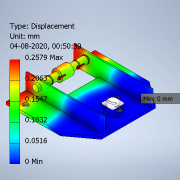
# Autodesk Inventor part: base for ball scew -bolt
Saved by Autodesk Inventor 2020 (Build 240168000, 168)
## iProperties
Created: 2020-07-27
Part Number: base for ball scew -bolt
Material: Steel, Mild
Document SubType Name: Modeling
Designer: Vikki
Mass: 4960.92 g
Surface Area: 1915.07 cm^2
Volume: 631.964 cm^3
Density: 7.85 g/cm^3
Appearance: Semi-Polished
Author: Vikki
Autodesk Inventor part; units mm, degrees
ref_plane "Work Plane1" through (0, 0, 4950) normal (0, 0, 1) x (1, 0, 0)
sketch "Sketch1" plane through (0, 0, 4950) normal (0, 0, 1) x (1, 0, 0)
  circle A0 centre (180, 0) radius 12.5 projected
  circle A1 centre (180, 17.5) radius 2 projected
  circle A2 centre (197.5, 0) radius 2 projected
  circle A3 centre (162.5, 0) radius 2 projected
  circle A4 centre (180, -17.5) radius 2 projected
  line L0 (40, 182.7) -> (-40, 182.7) projected
  line L1 (-40, 182.7) -> (-40, -182.7) projected
  line L2 (-40, -182.7) -> (40, -182.7) projected
  line L3 (40, -182.7) -> (40, -50) projected
  line L4 (40, -50) -> (260, -50) projected
  line L5 (260, -50) -> (260, 50) projected
  line L6 (260, 50) -> (40, 50) projected
  line L7 (40, 50) -> (40, 182.7) projected
  circle A5 centre (0, 120) radius 8 projected
  circle A6 centre (0, -120) radius 8 projected
  circle A7 centre (0, -120) radius 8.5
  circle A8 centre (0, 120) radius 8.5
  line L8 (40, 182.7) -> (40, -182.7)
  line L9 (40, -182.7) -> (80, -182.7)
  line L10 (80, -182.7) -> (80, 182.7)
  line L11 (80, 182.7) -> (40, 182.7)
  line L12 (-40, 75) -> (40, 75)
  line L13 (40, 75) -> (40, -75)
  line L14 (40, -75) -> (-40, -75)
  line L15 (80, 182.7) -> (260, 50)
  line L16 (260, -50) -> (80, -182.7)
  line L17 (80, -142.7) -> (-40, -142.7)
  line L18 (-40, 142.7) -> (80, 142.7)
  line L19 (80, 142.7) -> (134.2577, 142.7)
  line L20 (80, -142.7) -> (134.2577, -142.7)
  line L21 (210, 86.8611) -> (210, -86.8611)
  point P0 (0, 0)
  point P1 (40, 75)
  dimension "d0" = 17
  dimension "d1" = 17
  dimension "d2" = 40
  dimension "d3" = 40
  dimension "d4" = 75
  dimension "d5" = 75
  dimension "d23" = 40
  dimension "d24" = 40
  dimension "d25" = 50
  constraints: 28 end point, 10 point on line, 5 perpendicular, 4 parallel, 2 centre point, 2 coincident, 2 horizontal, 1 vertical
  measures "d0" diameter of A7
  measures "d1" diameter of A8
  measures "d2" distance of L2.end L9.end
  measures "d3" distance from line of point (0, 0) L13
  measures "d4" distance from line of point (0, 0) L14
  measures "d5" distance from line of L12 point (0, 0)
  measures "d23" distance between parallel lines of L17 L2
  measures "d24" distance between parallel lines of L0 L18
  measures "d25" distance between parallel lines of L21 L5
extrude "Extrusion1" add sketch "Sketch1" along normal blind 8 contours A0 | A1 | A2 | A3 | A4 | L18 L10 L6 L7 | L7 L12 L1 L18 | L19 L15 L21 L6 L10 | L6 L10 L4 L8 | L6 L21 L4 L10 | L14 L3 L17 L1 | L4 L10 L17 L3 | L4 L21 L16 L20 L10
sketch "Sketch2" plane through (0, 0, 4958) normal (0, 0, 1) x (1, 0, 0)
  line L0 (-40, 75) -> (40, 75) projected
  line L1 (-40, 75) -> (40, 75)
  line L2 (40, 75) -> (40, 79)
  line L3 (40, 79) -> (-40, 79)
  line L4 (-40, 79) -> (-40, 75)
  line L5 (40, -75) -> (-40, -75) projected
  line L6 (40, -75) -> (-40, -75)
  line L7 (-40, -75) -> (-40, -79)
  line L8 (-40, -79) -> (40, -79)
  line L9 (40, -79) -> (40, -75)
  line L10 (-20, 79) -> (-20, -79)
  line L11 (20, -79) -> (20, 79)
  point P0 (0, 0)
  point P1 (20, 75)
  point P2 (-20, 75)
  point P3 (20, -75)
  point P4 (-20, -75)
  dimension "d8" = 4
  dimension "d9" = 4
  dimension "d12" = 20
  dimension "d13" = 20
  constraints: 20 end point, 6 equal length, 4 perpendicular, 4 point on line
  measures "d8" distance of L0.end L2.end
  measures "d9" distance of L8.end L5.start
  measures "d12" distance from line of L10 point (0, 0)
  measures "d13" distance from line of L11 point (0, 0)
extrude "Extrusion2" add sketch "Sketch2" along normal blind 50 contours L10 L3 L11 L0 | L5 L11 L8 L10
sketch "Sketch3" plane through (-40, -75, 4950) normal (0, 1, 0) x (1, 0, 0)
  circle A0 centre (40, -38) radius 10.5
  line L0 (60, -58) -> (20, -58) projected
  line L1 (20, -8) -> (20, -58) projected
  point P0 (40, 4950)
  dimension "d16" = 21
  dimension "d17" = 20
  dimension "d18" = 20
  constraints: 1 centre point
  measures "d16" diameter of A0
  measures "d17" distance from line of L0 A0.centre
  measures "d18" distance from line of L1 A0.centre
extrude "Extrusion3" add sketch "Sketch3" along normal blind 163 and the other way blind 13
sketch "Sketch4" plane through (0, 0, 4958) normal (0, 0, 1) x (1, 0, 0)
  circle A0 centre (160, 17.5) radius 2 projected
  circle A1 centre (177.5, 0) radius 2 projected
  circle A2 centre (0, -120) radius 8 projected
  circle A3 centre (142.5, 0) radius 2 projected
  circle A4 centre (160, -17.5) radius 2 projected
  circle A5 centre (0, 120) radius 8 projected
  line L0 (30, 157.3) -> (30, 182.7) projected
  line L1 (40, 182.7) -> (30, 182.7) projected
  line L2 (40, 50) -> (40, 182.7) projected
  line L3 (260, 50) -> (40, 50) projected
  line L4 (260, -50) -> (260, 50) projected
  line L5 (40, -50) -> (260, -50) projected
  line L6 (40, -182.7) -> (40, -50) projected
  line L7 (30, -182.7) -> (40, -182.7) projected
  line L8 (30, -182.7) -> (30, -157.3) projected
  line L9 (30, -157.3) -> (-30, -157.3) projected
  line L10 (-30, -157.3) -> (-30, -182.7) projected
  line L11 (-40, -182.7) -> (-30, -182.7) projected
  line L12 (-40, 182.7) -> (-40, -182.7) projected
  line L13 (-30, 182.7) -> (-40, 182.7) projected
  line L14 (-30, 182.7) -> (-30, 157.3) projected
  line L15 (-30, 157.3) -> (30, 157.3) projected
  line L16 (250, 25.4) -> (224.6, 25.4) projected
  line L17 (224.6, 25.4) -> (224.6, -25.4) projected
  line L18 (224.6, -25.4) -> (250, -25.4) projected
  line L19 (250, -25.4) -> (250, 25.4) projected
  circle A6 centre (160, 0) radius 10 projected
  point P0 (0, 0)
extrude "Extrusion4" cut sketch "Sketch4" against normal up to surface (8 mm away) contours A0 | A1 | A3 | A4
sketch "Sketch5" plane through (0, 0, 4958) normal (0, 0, 1) x (1, 0, 0)
  circle A0 centre (160, 0) radius 7.5 projected
  circle A1 centre (160, 0) radius 8.25
  point P0 (0, 0)
  dimension "d28" = 16.5
  constraints: 1 centre point, 1 coincident
  measures "d28" diameter of A1
extrude "Extrusion5" cut sketch "Sketch5" against normal blind 10 contours A0 | A1
sketch "Sketch6" plane through (0, 0, 4950) normal (0, 0, -1) x (-1, 0, 0)
  circle A0 centre (-142.5, 0) radius 2 projected
  circle A1 centre (-177.5, 0) radius 2 projected
  circle A2 centre (-160, 17.5) radius 2 projected
  circle A3 centre (-160, -17.5) radius 2 projected
  line L0 (-134.2577, 142.7) -> (40, 142.7) projected
  line L1 (-210, 86.8611) -> (-134.2577, 142.7) projected
  line L2 (-210, -86.8611) -> (-210, 86.8611) projected
  line L3 (-134.2577, -142.7) -> (-210, -86.8611) projected
  line L4 (40, -142.7) -> (-134.2577, -142.7) projected
  line L5 (40, -75) -> (40, -142.7) projected
  line L6 (-40, -75) -> (40, -75) projected
  line L7 (-40, 75) -> (-40, -75) projected
  line L8 (40, 75) -> (-40, 75) projected
  line L9 (40, 142.7) -> (40, 75) projected
  circle A4 centre (0, -120) radius 8.5 projected
  circle A5 centre (0, 120) radius 8.5 projected
  circle A6 centre (-160, 0) radius 8.25 projected
  circle A7 centre (-160, 0) radius 22.5
  point P0 (0, 0)
  dimension "d31" = 45
  constraints: 1 centre point, 1 coincident
  measures "d31" diameter of A7
extrude "Extrusion6" add sketch "Sketch6" along normal blind 4 contours A7
sketch "Sketch7" plane through (160, 0, 4946) normal (0, 0, -1) x (-1, 0, 0)
  circle A0 centre (0, 0) radius 22.5 projected
  circle A1 centre (0, 0) radius 12.5
  circle A2 centre (0, 0) radius 9
  point P0 (160, 0)
  dimension "d34" = 25
  dimension "d47" = 18
  constraints: 2 centre point, 2 coincident
  measures "d34" diameter of A1
  measures "d47" diameter of A2
extrude "Extrusion7" add sketch "Sketch7" along normal blind 40 contours A1
sketch "Sketch9" plane through (0, 0, 5008) normal (0, 0, 1) x (1, 0, 0)
  circle A0 centre (160, 0) radius 8.25 construction
  circle A1 centre (142.5, 0) radius 2 construction
  circle A2 centre (177.5, 0) radius 2 construction
  circle A3 centre (160, 17.5) radius 2 construction
  circle A4 centre (160, -17.5) radius 2 construction
  line L0 (20, 79) -> (20, 75) projected
  line L1 (20, 75) -> (40, 75) projected
  line L2 (40, 75) -> (40, -75) projected
  line L3 (40, -75) -> (20, -75) projected
  line L4 (20, -75) -> (20, -79) projected
  line L5 (20, -79) -> (-20, -79) projected
  line L6 (-20, -79) -> (-20, -75) projected
  line L7 (-20, -75) -> (-40, -75) projected
  line L8 (-40, -75) -> (-40, -142.7) projected
  line L9 (-40, -142.7) -> (134.2577, -142.7) projected
  line L10 (134.2577, -142.7) -> (210, -86.8611) projected
  line L11 (210, -86.8611) -> (210, 86.8611) projected
  line L12 (210, 86.8611) -> (134.2577, 142.7) projected
  line L13 (134.2577, 142.7) -> (-40, 142.7) projected
  line L14 (-40, 142.7) -> (-40, 75) projected
  line L15 (-40, 75) -> (-20, 75) projected
  line L16 (-20, 75) -> (-20, 79) projected
  line L17 (-20, 79) -> (20, 79) projected
  circle A5 centre (0, -120) radius 8.5 projected
  circle A6 centre (0, 120) radius 8.5 projected
  circle A7 centre (160, 0) radius 12.5 projected
  circle A8 centre (160, 0) radius 9
  line L18 (20, -75) -> (-20, -75) projected
  line L19 (-20, 75) -> (20, 75) projected
  point P0 (0, 0)
  dimension "d37" = 18
  constraints: 1 centre point, 1 coincident
  measures "d37" diameter of A8
extrude "Extrusion8" [suppressed]
sketch "Sketch10" plane through (0, 0, 5012) normal (0, 0, 1) x (1, 0, 0)
  circle A0 centre (120, -75) radius 6
  circle A1 centre (90, 0) radius 6
  circle A2 centre (120, 75) radius 6
  circle A3 centre (160, 0) radius 12.5 projected
  point P0 (0, 0)
  dimension "d40" = 70
  dimension "d41" = 75
  dimension "d42" = 75
  dimension "d43" = 40
  dimension "d44" = 12
  constraints: 3 centre point, 2 equal radius, 1 horizontal alignment, 1 vertical alignment
  measures "d40" distance of A3.centre A1.centre
  measures "d41" vertical distance of A0.centre A3.centre
  measures "d42" vertical distance of A2.centre A3.centre
  measures "d43" horizontal distance of A3.centre A0.centre
  measures "d44" diameter of A0
extrude "Extrusion9" [suppressed]
sketch "Sketch11" plane through (20, -79, 4958) normal (1, 0, 0) x (0, 0, -1)
  line L0 (0, 4) -> (0, 0) projected
  line L1 (0, 4) -> (-50, 4) projected
  line L2 (-50, 0) -> (-50, 4) projected
  line L3 (0, 0) -> (-50, 0) projected
  line L4 (0, 158) -> (0, 154) projected
  line L5 (0, 158) -> (-50, 158) projected
  line L6 (-50, 154) -> (-50, 158) projected
  line L7 (0, 154) -> (-50, 154) projected
  point P0 (4958, 79)
extrude "Extrusion10" add sketch "Sketch11" along normal blind 190
sketch "Sketch12" plane through (-20, -79, 4958) normal (-1, 0, 0) x (0, 0, 1)
  line L0 (0, 154) -> (0, 158) projected
  line L1 (0, 154) -> (50, 154) projected
  line L2 (50, 158) -> (50, 154) projected
  line L3 (0, 158) -> (50, 158) projected
  line L4 (0, 0) -> (0, 4) projected
  line L5 (0, 0) -> (50, 0) projected
  line L6 (50, 4) -> (50, 0) projected
  line L7 (0, 4) -> (50, 4) projected
  point P0 (-4958, 79)
extrude "Extrusion11" add sketch "Sketch12" along normal up to surface (20 mm away)
ref_plane "Work Plane2" through (0, 0, 4954) normal (0, 0, 1) x (1, 0, 0)
mirror "Mirror1" about plane through (0, 0, 4954) normal (0, 0, 1) of "Extrusion6", "Extrusion7"
sketch "Sketch13" plane through (160, 0, 4906) normal (0, 0, -1) x (-1, 0, 0)
  circle A0 centre (0, 0) radius 9 projected
  circle A1 centre (4, 28) radius 75.6042
  point P0 (160, 0)
  constraints: 1 centre point
extrude "Extrusion12" cut sketch "Sketch13" against normal up to surface (44 mm away)
ref_plane "Work Plane3" through (-40, 73, 4950) normal (0, -1, 0) x (1, 0, 0)
sketch "Sketch14" plane through (-40, 73, 4950) normal (0, -1, 0) x (1, 0, 0)
  circle A0 centre (40, 38) radius 10.5 projected
  line L0 (0, 8) -> (250, 8) projected
  line L1 (0, 8) -> (0, 58) projected
  line L2 (0, 58) -> (250, 58) projected
  line L3 (250, 8) -> (250, 58) projected
  circle A1 centre (40, 38) radius 12
  point P0 (40, -4950)
  dimension "d55" = 24
  constraints: 1 centre point, 1 coincident
  measures "d55" diameter of A1
extrude "Extrusion13" add sketch "Sketch14" along normal blind 2 contours A1
mirror "Mirror2" about plane through (0, 0, 0) normal (0, 1, 0) of "Extrusion13"
ref_plane "Work Plane4" through (-40, 0, 4950) normal (0, 1, 0) x (1, 0, 0)
sketch "Sketch15" plane through (-40, 0, 4950) normal (0, 1, 0) x (1, 0, 0)
  circle A0 centre (40, -38) radius 10.5 projected
  circle A1 centre (40, -38) radius 10.5 projected
  circle A2 centre (40, -38) radius 17.5
  point P0 (40, 4950)
  dimension "d58" = 35
  constraints: 1 centre point, 1 coincident
  measures "d58" diameter of A2
extrude "Extrusion14" add sketch "Sketch15" along normal mid plane 37
pattern_linear "Rectangular Pattern1" count 2 spacing 29 along (0, -1, 0) of "Extrusion13"
mirror "Mirror3" about plane through (0, 0, 0) normal (0, 1, 0) of "Extrusion13", "Rectangular Pattern1"
equation "\"d4\" = d5"
equation "\"d8\" = d9"
body "Solid1"
